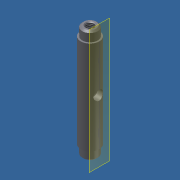
# Autodesk Inventor part: EIXO DIANTEIRO(34)
Saved by Autodesk Inventor 2012 SP1 (Build 160190100, 190)
## iProperties
Created: 2012-07-23
Part Number: EIXO DIANTEIRO(34)
Material: Carbon Steel
Document SubType Name: Modeling
Designer: bruno.silveira
Mass: 363.942 g
Surface Area: 119.632 cm^2
Volume: 46.2442 cm^3
Density: 7.87 g/cm^3
Author: bruno.silveira
Autodesk Inventor part; units mm, degrees
ref_plane "XZ Plane" through (0, 0, 0) normal (0, 1, 0) x (-1, 0, 0)
ref_plane "XY Plane" through (0, 0, 0) normal (0, 0, 1) x (1, 0, 0)
sketch "Sketch1" plane through (0, 0, 0) normal (0, 0, 1) x (1, 0, 0)
  circle A0 centre (0, 0) radius 8
  dimension "d0" = 16
  constraints: 1 centre point, 1 coincident
  measures "d0" diameter of A0
extrude "Extrusion1" add sketch "Sketch1" along normal blind 73
sketch "Sketch2" plane through (0, 0, 0) normal (0, 0, -1) x (-1, 0, 0)
  circle A0 centre (0, 0) radius 8 projected
  circle A1 centre (0, 0) radius 5
  dimension "d6" = 10
  constraints: 1 centre point, 1 coincident
  measures "d6" diameter of A1
extrude "Extrusion2" cut sketch "Sketch2" against normal blind 6.2
sketch "Sketch3" plane through (0, 0, 73) normal (0, 0, 1) x (1, 0, 0)
  circle A0 centre (0, 0) radius 8 projected
  circle A1 centre (0, 0) radius 5
  dimension "d9" = 10
  constraints: 1 centre point, 1 coincident
  measures "d9" diameter of A1
extrude "Extrusion3" cut sketch "Sketch3" against normal blind 6.2
chamfer "Chamfer2" distance 1 angle 45 2 edges at (-5, 0, 73) (5, 0, 0)
sketch "Sketch4" plane through (0, 0, 0) normal (0, 0, -1) x (-1, 0, 0)
  circle A0 centre (0, 0) radius 4 projected
  constraints: 1 coincident
hole "Hole1" at (0, 0, 0) direction (0, 0, 1) diameter 4.917 depth 12 tip angle 118 thread size "M6x1" class "6H" standard "ANSI Metric M Profile"
sketch "Sketch5" plane through (0, 0, 73) normal (0, 0, 1) x (1, 0, 0)
  circle A0 centre (0, 0) radius 4 projected
  constraints: 1 coincident
hole "Hole2" at (0, 0, 73) direction (0, 0, -1) diameter 4.917 depth 12 tip angle 118 thread size "M6x1" class "6H" standard "ANSI Metric M Profile"
chamfer "Chamfer3" distance 0.5 angle 45 2 edges at (0, 2.4585, 73) (0, -2.4585, 0)
sketch "Sketch6" plane through (0, 0, 66.8) normal (0, 0, 1) x (1, 0, 0)
  circle A0 centre (0, 0) radius 8 projected
  circle A1 centre (0, 0) radius 6
  dimension "d32" = 12
  constraints: 1 centre point, 1 coincident
  measures "d32" diameter of A1
extrude "Extrusion4" cut sketch "Sketch6" against normal blind 60.6
ref_plane "Work Plane1" through (6, 0, 66.8) normal (1, 0, 0) x (0, 1, 0)
sketch "Sketch7" plane through (6, 0, 66.8) normal (1, 0, 0) x (0, 1, 0)
  line L0 (-6, -60.6) -> (6, -60.6) projected
  line L1 (6, 0) -> (-6, 0) projected
  circle A0 centre (0, -30.3) radius 3
  point P0 (0, -66.8)
  dimension "d35" = 6
  dimension "d36" = 30.3
  constraints: 1 centre point
  measures "d35" diameter of A0
  measures "d36" distance from line of L1 A0.centre
hole "Hole3" at (6, 0, 36.5) direction (-1, 0, 0) diameter 6 depth 4 tip angle 118
body "Solid1"
